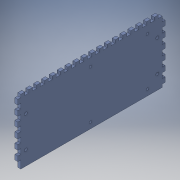
# Autodesk Inventor part: 000.202 - Боковая стенка пустая
Saved by Autodesk Inventor 2019 (Build 230136000, 136)
## iProperties
Created: 2020-02-27
Part Number: 000.202 - Боковая стенка пустая
Material: Пластик АБС
Document SubType Name: Modeling
Designer: Петров Иван
Density: 1.06 g/cm^3
Appearance: Резина — синяя
Author: Петров Иван
Autodesk Inventor part; units mm, degrees
ref_plane "YZ Plane" through (0, 0, 0) normal (1, 0, 0) x (0, 1, 0)
ref_plane "XZ Plane" through (0, 0, 0) normal (0, 1, 0) x (-1, 0, 0)
ref_plane "XY Plane" through (0, 0, 0) normal (0, 0, 1) x (1, 0, 0)
sketch "Эскиз1" plane through (0, 0, 0) normal (1, 0, 0) x (0, 1, 0)
  line L0 (-32.5, 72) -> (32.5, 72)
  line L1 (32.5, 72) -> (32.5, -72)
  line L2 (32.5, -72) -> (-32.5, -72)
  line L3 (-32.5, -72) -> (-32.5, 72)
  line L4 (-32.5, 72) -> (32.5, -72) construction
  line L5 (32.5, 72) -> (-32.5, -72) construction
  point P0 (0, 0)
  dimension "d0" = 65
  dimension "d1" = 144
  constraints: 12 end point, 2 midpoint, 2 parallel, 1 horizontal, 1 perpendicular
  measures "d0" distance of L1.end L2.end
  measures "d1" distance of L0.end L1.end
extrude "Выдавливание1" add sketch "Эскиз1" along normal blind 3
sketch "Эскиз2" plane through (3, 0, 0) normal (1, 0, 0) x (0, 0, -1)
  line L0 (-72, -32.5) -> (72, -32.5) projected
  line L1 (-72, -32.5) -> (-68, -32.5)
  line L2 (-68, -32.5) -> (-68, -35.5)
  line L3 (-68, -35.5) -> (-72, -35.5)
  line L4 (-72, -35.5) -> (-72, -32.5)
  point P0 (0, 0)
  dimension "d4" = 4
  dimension "d5" = 3
  constraints: 8 end point, 2 parallel, 1 horizontal, 1 perpendicular
  measures "d4" distance of L2.end L3.end
  measures "d5" distance of L1.end L2.end
extrude "Выдавливание2" add sketch "Эскиз2" against normal blind 3
pattern_linear "Прямоуг.массив1" count 18 spacing 8 along (0, 0, -1) of "Выдавливание2"
sketch "Эскиз3" plane through (3, 0, 0) normal (1, 0, 0) x (0, 0, -1)
  line L0 (72, 32.5) -> (-72, 32.5) projected
  line L1 (-72, 32.5) -> (-75, 32.5)
  line L2 (-75, 32.5) -> (-75, 27.5)
  line L3 (-75, 27.5) -> (-72, 27.5)
  line L4 (-72, 27.5) -> (-72, 32.5)
  line L5 (72, -32.5) -> (72, 32.5) projected
  line L6 (72, 27.5) -> (75, 27.5)
  line L7 (75, 27.5) -> (75, 22.5)
  line L8 (75, 22.5) -> (72, 22.5)
  line L9 (72, 22.5) -> (72, 27.5)
  point P0 (0, 0)
  dimension "d11" = 3
  dimension "d12" = 5
  dimension "d13" = 3
  dimension "d14" = 5
  dimension "d15" = 5
  constraints: 16 end point, 4 parallel, 2 horizontal, 2 perpendicular, 1 point on line
  measures "d11" distance of L3.end L2.end
  measures "d12" distance of L2.end L1.end
  measures "d13" distance of L7.end L8.end
  measures "d14" distance of L6.end L7.end
  measures "d15" distance between parallel lines of L0 L6
extrude "Выдавливание3" add sketch "Эскиз3" against normal blind 3
pattern_linear "Прямоуг.массив2" count 6 spacing 10 along (0, -1, 0) of "Выдавливание3"
mirror "Зеркальное отражение1" about plane through (0, 0, 0) normal (0, 1, 0) of "Выдавливание2", "Прямоуг.массив1"
sketch "Эскиз4" plane through (0, 0, 0) normal (-1, 0, 0) x (0, 0, 1)
  line L0 (-24.49, 2.034) -> (-35.69, 2.034) projected
  line L1 (-24.49, 2.034) -> (-24.49, -7.766) projected
  line L2 (-35.69, 2.034) -> (-35.69, -7.766) projected
  line L3 (-35.69, -8.166) -> (-24.49, -8.166) projected
  line L4 (-35.69, -7.766) -> (-35.69, -8.166) projected
  line L5 (-24.49, -8.166) -> (-24.49, -7.766) projected
  line L6 (34.27, -8.7) -> (18.25, -8.7) projected
  line L7 (18.25, -8.7) -> (18.25, 6.6) projected
  line L8 (34.27, 6.6) -> (18.25, 6.6) projected
  line L9 (34.27, -8.7) -> (34.27, 6.6) projected
  line L10 (38.35, 6.5) -> (38.35, -8.7) projected
  line L11 (51.25, 6.5) -> (38.75, 6.5) projected
  line L12 (69.65, -8.7) -> (69.65, 6.5) projected
  line L13 (38.35, 6.5) -> (69.65, 6.5)
  line L14 (69.65, 6.5) -> (69.65, -8.7)
  line L15 (69.65, -8.7) -> (38.35, -8.7)
  line L16 (38.35, -8.7) -> (38.35, 6.5)
  point P0 (0, 0)
  dimension "d23" = 0
  constraints: 8 end point, 2 parallel, 1 horizontal, 1 perpendicular
  measures "d23" distance between parallel lines of L12 L14
extrude "Выдавливание4" [suppressed]
sketch "Эскиз5" plane through (3, 35.5, -64) normal (0, 1, 0) x (1, 0, 0)
  line L0 (0, 4) -> (0, 8) projected
  line L1 (-3, -56) -> (-3, -60) projected
  line L2 (0, 4) -> (-3, 4)
  line L3 (-3, 4) -> (-3, -56)
  line L4 (-3, -56) -> (0, -56)
  line L5 (0, -56) -> (0, 4)
  point P0 (-3, -64)
  constraints: 8 end point, 2 parallel, 1 horizontal, 1 perpendicular
extrude "Выдавливание5" [suppressed]
sketch "Эскиз7" plane through (3, 0, 0) normal (1, 0, 0) x (0, 0, -1)
  line L0 (-75, -17.5) -> (-75, -22.5) projected
  line L1 (-75, -22.5) -> (-75, -35.5)
  line L2 (-75, -35.5) -> (75, -35.5)
  line L3 (75, -35.5) -> (75, -30.5)
  line L4 (75, -30.5) -> (-75, -30.5)
  line L5 (-75, -30.5) -> (-75, -35.5)
  line L6 (-72, -22.5) -> (-72, -35.5) projected
  line L7 (-72, 27.5) -> (-72, 22.5) projected
  line L8 (-72, 22.5) -> (-75, 22.5) projected
  line L9 (-75, 22.5) -> (-75, 17.5) projected
  line L10 (-75, 17.5) -> (-72, 17.5) projected
  line L11 (-72, 17.5) -> (-72, 12.5) projected
  line L12 (-72, 12.5) -> (-75, 12.5) projected
  line L13 (-75, 12.5) -> (-75, 7.5) projected
  line L14 (-75, 7.5) -> (-72, 7.5) projected
  line L15 (-72, 7.5) -> (-72, 2.5) projected
  line L16 (-72, 2.5) -> (-75, 2.5) projected
  line L17 (-75, 2.5) -> (-75, -2.5) projected
  line L18 (-75, -2.5) -> (-72, -2.5) projected
  line L19 (-72, -2.5) -> (-72, -7.5) projected
  line L20 (-72, -7.5) -> (-75, -7.5) projected
  line L21 (-75, -7.5) -> (-75, -12.5) projected
  line L22 (-75, -12.5) -> (-72, -12.5) projected
  line L23 (-72, -12.5) -> (-72, -17.5) projected
  line L24 (-72, -17.5) -> (-75, -17.5) projected
  line L25 (-75, -17.5) -> (-75, -22.5) projected
  line L26 (-75, -22.5) -> (-72, -22.5) projected
  line L27 (-72, -22.5) -> (-72, -35.5) projected
  line L28 (-68, -35.5) -> (-72, -35.5) projected
  line L29 (-68, -32.5) -> (-68, -35.5) projected
  line L30 (-68, -32.5) -> (-64, -32.5) projected
  line L31 (-64, -35.5) -> (-64, -32.5) projected
  line L32 (-60, -35.5) -> (-64, -35.5) projected
  line L33 (-60, -32.5) -> (-60, -35.5) projected
  line L34 (-60, -32.5) -> (-56, -32.5) projected
  line L35 (-56, -35.5) -> (-56, -32.5) projected
  line L36 (-52, -35.5) -> (-56, -35.5) projected
  line L37 (-52, -32.5) -> (-52, -35.5) projected
  line L38 (-52, -32.5) -> (-48, -32.5) projected
  line L39 (-48, -35.5) -> (-48, -32.5) projected
  line L40 (-44, -35.5) -> (-48, -35.5) projected
  line L41 (-44, -32.5) -> (-44, -35.5) projected
  line L42 (-44, -32.5) -> (-40, -32.5) projected
  line L43 (-40, -35.5) -> (-40, -32.5) projected
  line L44 (-36, -35.5) -> (-40, -35.5) projected
  line L45 (-36, -32.5) -> (-36, -35.5) projected
  line L46 (-36, -32.5) -> (-32, -32.5) projected
  line L47 (-32, -35.5) -> (-32, -32.5) projected
  line L48 (-28, -35.5) -> (-32, -35.5) projected
  line L49 (-28, -32.5) -> (-28, -35.5) projected
  line L50 (-28, -32.5) -> (-24, -32.5) projected
  line L51 (-24, -35.5) -> (-24, -32.5) projected
  line L52 (-20, -35.5) -> (-24, -35.5) projected
  line L53 (-20, -32.5) -> (-20, -35.5) projected
  line L54 (-20, -32.5) -> (-16, -32.5) projected
  line L55 (-16, -35.5) -> (-16, -32.5) projected
  line L56 (-12, -35.5) -> (-16, -35.5) projected
  line L57 (-12, -32.5) -> (-12, -35.5) projected
  line L58 (-12, -32.5) -> (-8, -32.5) projected
  line L59 (-8, -35.5) -> (-8, -32.5) projected
  line L60 (-4, -35.5) -> (-8, -35.5) projected
  line L61 (-4, -32.5) -> (-4, -35.5) projected
  line L62 (-4, -32.5) -> (0, -32.5) projected
  line L63 (0, -35.5) -> (0, -32.5) projected
  line L64 (4, -35.5) -> (0, -35.5) projected
  line L65 (4, -32.5) -> (4, -35.5) projected
  line L66 (4, -32.5) -> (8, -32.5) projected
  line L67 (8, -35.5) -> (8, -32.5) projected
  line L68 (12, -35.5) -> (8, -35.5) projected
  line L69 (12, -32.5) -> (12, -35.5) projected
  line L70 (12, -32.5) -> (16, -32.5) projected
  line L71 (16, -35.5) -> (16, -32.5) projected
  line L72 (20, -35.5) -> (16, -35.5) projected
  line L73 (20, -32.5) -> (20, -35.5) projected
  line L74 (20, -32.5) -> (24, -32.5) projected
  line L75 (24, -35.5) -> (24, -32.5) projected
  line L76 (28, -35.5) -> (24, -35.5) projected
  line L77 (28, -32.5) -> (28, -35.5) projected
  line L78 (28, -32.5) -> (32, -32.5) projected
  line L79 (32, -35.5) -> (32, -32.5) projected
  line L80 (36, -35.5) -> (32, -35.5) projected
  line L81 (36, -32.5) -> (36, -35.5) projected
  line L82 (36, -32.5) -> (40, -32.5) projected
  line L83 (40, -35.5) -> (40, -32.5) projected
  line L84 (44, -35.5) -> (40, -35.5) projected
  line L85 (44, -32.5) -> (44, -35.5) projected
  line L86 (44, -32.5) -> (48, -32.5) projected
  line L87 (48, -35.5) -> (48, -32.5) projected
  line L88 (52, -35.5) -> (48, -35.5) projected
  line L89 (52, -32.5) -> (52, -35.5) projected
  line L90 (52, -32.5) -> (56, -32.5) projected
  line L91 (56, -35.5) -> (56, -32.5) projected
  line L92 (60, -35.5) -> (56, -35.5) projected
  line L93 (60, -32.5) -> (60, -35.5) projected
  line L94 (60, -32.5) -> (64, -32.5) projected
  line L95 (64, -35.5) -> (64, -32.5) projected
  line L96 (68, -35.5) -> (64, -35.5) projected
  line L97 (68, -32.5) -> (68, -35.5) projected
  line L98 (68, -32.5) -> (72, -32.5) projected
  line L99 (72, -32.5) -> (72, -27.5) projected
  line L100 (72, -27.5) -> (75, -27.5) projected
  line L101 (75, -27.5) -> (75, -22.5) projected
  line L102 (75, -22.5) -> (72, -22.5) projected
  line L103 (72, -22.5) -> (72, -17.5) projected
  line L104 (72, -17.5) -> (75, -17.5) projected
  line L105 (75, -17.5) -> (75, -12.5) projected
  line L106 (75, -12.5) -> (72, -12.5) projected
  line L107 (72, -12.5) -> (72, -7.5) projected
  line L108 (72, -7.5) -> (75, -7.5) projected
  line L109 (75, -7.5) -> (75, -2.5) projected
  line L110 (75, -2.5) -> (72, -2.5) projected
  line L111 (72, -2.5) -> (72, 2.5) projected
  line L112 (72, 2.5) -> (75, 2.5) projected
  line L113 (75, 2.5) -> (75, 7.5) projected
  line L114 (75, 7.5) -> (72, 7.5) projected
  line L115 (72, 7.5) -> (72, 12.5) projected
  line L116 (72, 12.5) -> (75, 12.5) projected
  line L117 (75, 12.5) -> (75, 17.5) projected
  line L118 (75, 17.5) -> (72, 17.5) projected
  line L119 (72, 17.5) -> (72, 22.5) projected
  line L120 (72, 22.5) -> (75, 22.5) projected
  line L121 (75, 22.5) -> (75, 27.5) projected
  line L122 (75, 27.5) -> (72, 27.5) projected
  line L123 (72, 27.5) -> (72, 32.5) projected
  line L124 (72, 32.5) -> (68, 32.5) projected
  line L125 (68, 32.5) -> (68, 35.5) projected
  line L126 (68, 35.5) -> (64, 35.5) projected
  line L127 (64, 35.5) -> (64, 32.5) projected
  line L128 (64, 32.5) -> (60, 32.5) projected
  line L129 (60, 32.5) -> (60, 35.5) projected
  line L130 (60, 35.5) -> (56, 35.5) projected
  line L131 (56, 35.5) -> (56, 32.5) projected
  line L132 (56, 32.5) -> (52, 32.5) projected
  line L133 (52, 32.5) -> (52, 35.5) projected
  line L134 (52, 35.5) -> (48, 35.5) projected
  line L135 (48, 35.5) -> (48, 32.5) projected
  line L136 (48, 32.5) -> (44, 32.5) projected
  line L137 (44, 32.5) -> (44, 35.5) projected
  line L138 (44, 35.5) -> (40, 35.5) projected
  line L139 (40, 35.5) -> (40, 32.5) projected
  line L140 (40, 32.5) -> (36, 32.5) projected
  line L141 (36, 32.5) -> (36, 35.5) projected
  line L142 (36, 35.5) -> (32, 35.5) projected
  line L143 (32, 35.5) -> (32, 32.5) projected
  line L144 (32, 32.5) -> (28, 32.5) projected
  line L145 (28, 32.5) -> (28, 35.5) projected
  line L146 (28, 35.5) -> (24, 35.5) projected
  line L147 (24, 35.5) -> (24, 32.5) projected
  line L148 (24, 32.5) -> (20, 32.5) projected
  line L149 (20, 32.5) -> (20, 35.5) projected
  line L150 (20, 35.5) -> (16, 35.5) projected
  line L151 (16, 35.5) -> (16, 32.5) projected
  line L152 (16, 32.5) -> (12, 32.5) projected
  line L153 (12, 32.5) -> (12, 35.5) projected
  line L154 (12, 35.5) -> (8, 35.5) projected
  line L155 (8, 35.5) -> (8, 32.5) projected
  line L156 (8, 32.5) -> (4, 32.5) projected
  line L157 (4, 32.5) -> (4, 35.5) projected
  line L158 (4, 35.5) -> (0, 35.5) projected
  line L159 (0, 35.5) -> (0, 32.5) projected
  line L160 (0, 32.5) -> (-4, 32.5) projected
  line L161 (-4, 32.5) -> (-4, 35.5) projected
  line L162 (-4, 35.5) -> (-8, 35.5) projected
  line L163 (-8, 35.5) -> (-8, 32.5) projected
  line L164 (-8, 32.5) -> (-12, 32.5) projected
  line L165 (-12, 32.5) -> (-12, 35.5) projected
  line L166 (-12, 35.5) -> (-16, 35.5) projected
  line L167 (-16, 35.5) -> (-16, 32.5) projected
  line L168 (-16, 32.5) -> (-20, 32.5) projected
  line L169 (-20, 32.5) -> (-20, 35.5) projected
  line L170 (-20, 35.5) -> (-24, 35.5) projected
  line L171 (-24, 35.5) -> (-24, 32.5) projected
  line L172 (-24, 32.5) -> (-28, 32.5) projected
  line L173 (-28, 32.5) -> (-28, 35.5) projected
  line L174 (-28, 35.5) -> (-32, 35.5) projected
  line L175 (-32, 35.5) -> (-32, 32.5) projected
  line L176 (-32, 32.5) -> (-36, 32.5) projected
  line L177 (-36, 32.5) -> (-36, 35.5) projected
  line L178 (-36, 35.5) -> (-40, 35.5) projected
  line L179 (-40, 35.5) -> (-40, 32.5) projected
  line L180 (-40, 32.5) -> (-44, 32.5) projected
  line L181 (-44, 32.5) -> (-44, 35.5) projected
  line L182 (-44, 35.5) -> (-48, 35.5) projected
  line L183 (-48, 35.5) -> (-48, 32.5) projected
  line L184 (-48, 32.5) -> (-52, 32.5) projected
  line L185 (-52, 32.5) -> (-52, 35.5) projected
  line L186 (-52, 35.5) -> (-56, 35.5) projected
  line L187 (-56, 35.5) -> (-56, 32.5) projected
  line L188 (-56, 32.5) -> (-60, 32.5) projected
  line L189 (-60, 32.5) -> (-60, 35.5) projected
  line L190 (-60, 35.5) -> (-64, 35.5) projected
  line L191 (-64, 35.5) -> (-64, 32.5) projected
  line L192 (-64, 32.5) -> (-68, 32.5) projected
  line L193 (-68, 32.5) -> (-68, 35.5) projected
  line L194 (-68, 35.5) -> (-72, 35.5) projected
  line L195 (-72, 35.5) -> (-72, 32.5) projected
  line L196 (-72, 32.5) -> (-75, 32.5) projected
  line L197 (-75, 32.5) -> (-75, 27.5) projected
  line L198 (-75, 27.5) -> (-72, 27.5) projected
  point P0 (0, 0)
  dimension "d31" = 5
  constraints: 10 end point, 2 parallel, 1 horizontal, 1 perpendicular, 1 vertical
  measures "d31" distance of L3.end L2.end
extrude "Выдавливание7" cut sketch "Эскиз7" against normal blind 10 contours L4 L6 L2 L1 | L4 L99 L98 L97 L2 L95 L94 L93 L91 L90 L89 L87 L86 L85 L83 L82 L81 L79 L78 L77 L75 L74 L73 L71 L70 L69 L67 L66 L65 L63 L62 L61 L59 L58 L57 L55 L54 L53 L51 L50 L49 L47 L46 L45 L43 L42 L41 L39 L38 L37 L35 L34 L33 L31 L30 L29 L6 | L4 L3 L2 L97 L98 L99 | L29 L30 L31 L2 | L33 L34 L35 L2 | L2 L93 L94 L95 | L37 L38 L39 L2 | L2 L89 L90 L91 | L41 L42 L43 L2 | L2 L85 L86 L87 | L45 L46 L47 L2 | L2 L81 L82 L83 | L49 L50 L51 L2 | L2 L77 L78 L79 | L53 L54 L55 L2 | L2 L73 L74 L75 | L57 L58 L59 L2 | L2 L69 L70 L71 | L61 L62 L63 L2 | L2 L65 L66 L67
sketch "Эскиз9" plane through (0, 0, 0) normal (-1, 0, 0) x (0, 0, 1)
  circle A0 centre (-67, -16) radius 1.5
  circle A1 centre (-67, 16) radius 1.5
  line L0 (-62, 20) -> (-72, 20)
  line L1 (-72, 20) -> (-72, -20)
  line L2 (-72, -20) -> (-62, -20)
  line L3 (-62, -20) -> (-62, 20)
  line L4 (-72, 2.5) -> (-72, -2.5) projected
  line L5 (-72, 20) -> (-62, -20) construction
  line L6 (-72, -20) -> (-62, 20) construction
  point P0 (-67, 0)
  dimension "d45" = 5
  dimension "d46" = 4
  dimension "d47" = 5
  dimension "d48" = 5
  dimension "d49" = 4
  dimension "d50" = 5
  dimension "d51" = 5
  constraints: 12 end point, 2 centre point, 1 midpoint
  measures "d45" distance from line of L4 point (-67, 0)
  measures "d46" distance from line of L0 A1.centre
  measures "d47" distance from line of L3 A1.centre
  measures "d48" distance from line of L3 A0.centre
  measures "d49" distance from line of L2 A0.centre
  measures "d50" distance from line of L1 A0.centre
  measures "d51" distance from line of L1 A1.centre
extrude "Выдавливание9" cut sketch "Эскиз9" against normal blind 10 contours A0 | A1
mirror "Зеркальное отражение3" about plane through (0, 0, 0) normal (0, 0, 1) of "Выдавливание9"
sketch "Эскиз10" plane through (3, 0, 0) normal (1, 0, 0) x (0, 0, -1)
  line L0 (60.3747, 25.4747) -> (60.3747, -25.5253)
  arc A0 (60.3747, 25.4747) -> (57.8747, 27.9747) centre (57.8747, 25.4747) ccw
  line L1 (-22.1253, 27.9747) -> (57.8747, 27.9747)
  arc A1 (-22.1253, 27.9747) -> (-24.6253, 25.4747) centre (-22.1253, 25.4747) ccw
  line L2 (-24.6253, -25.5253) -> (-24.6253, 25.4747)
  arc A2 (-24.6253, -25.5253) -> (-22.1253, -28.0253) centre (-22.1253, -25.5253) ccw
  line L3 (57.8747, -28.0253) -> (-22.1253, -28.0253)
  arc A3 (57.8747, -28.0253) -> (60.3747, -25.5253) centre (57.8747, -25.5253) ccw
  circle A4 centre (56.8747, 24.4747) radius 1.25
  circle A5 centre (56.8747, -24.5253) radius 1.25
  circle A6 centre (-1.1253, -24.5253) radius 1.25
  circle A7 centre (-1.1253, 24.4747) radius 1.25
  point P0 (17.8747, -0.0253)
  constraints: 8 centre point, 8 end point, 8 point on circle
extrude "Выдавливание10" cut sketch "Эскиз10" against normal blind 10 contours A4 | A5 | A6 | A7
